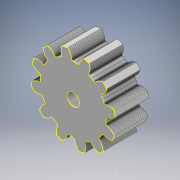
# Autodesk Inventor part: Engranaje_V_P_2
Saved by Autodesk Inventor 2017 (Build 210142000, 142)
## iProperties
Created: 2016-10-02
Part Number: Engranaje_V_P_2
Material: Generic
Document SubType Name: Modeling
Designer: CASA
Density: 1 g/cm^3
Appearance: Default
Author: CASA
Autodesk Inventor part; units mm, degrees
(part 1 of 2)
ref_plane "YZ Plane" through (0, 0, 0) normal (1, 0, 0) x (0, 1, 0)
ref_plane "XZ Plane" through (0, 0, 0) normal (0, 1, 0) x (-1, 0, 0)
ref_plane "XY Plane" through (0, 0, 0) normal (0, 0, 1) x (1, 0, 0)
sketch "Sketch1" plane through (0, 0, 0) normal (0, 1, 0) x (-1, 0, 0)
  line L0 (0.4524, 0.3799) -> (0.4499, 0.3611)
  line L1 (0.4499, 0.3611) -> (0.4427, 0.3436)
  line L2 (0.4427, 0.3436) -> (0.4311, 0.3286)
  line L3 (0.4311, 0.3286) -> (0.4161, 0.3171)
  line L4 (0.4161, 0.3171) -> (0.3986, 0.3099)
  line L5 (0.3986, 0.3099) -> (0.3799, 0.3074)
  line L6 (0.3799, 0.3074) -> (0.3611, 0.3099)
  line L7 (0.3611, 0.3099) -> (0.3436, 0.3171)
  line L8 (0.3436, 0.3171) -> (0.3286, 0.3286)
  line L9 (0.3286, 0.3286) -> (0.3171, 0.3436)
  line L10 (0.3171, 0.3436) -> (0.3099, 0.3611)
  line L11 (0.3099, 0.3611) -> (0.3074, 0.3799)
  line L12 (0.3074, 0.3799) -> (0.3099, 0.3987)
  line L13 (0.3099, 0.3987) -> (0.3171, 0.4161)
  line L14 (0.3171, 0.4161) -> (0.3286, 0.4312)
  line L15 (0.3286, 0.4312) -> (0.3436, 0.4427)
  line L16 (0.3436, 0.4427) -> (0.3611, 0.4499)
  line L17 (0.3611, 0.4499) -> (0.3799, 0.4524)
  line L18 (0.3799, 0.4524) -> (0.3987, 0.4499)
  line L19 (0.3987, 0.4499) -> (0.4161, 0.4427)
  line L20 (0.4161, 0.4427) -> (0.4312, 0.4312)
  line L21 (0.4312, 0.4312) -> (0.4427, 0.4161)
  line L22 (0.4427, 0.4161) -> (0.4499, 0.3987)
  line L23 (0.4499, 0.3987) -> (0.4524, 0.3799)
  line L24 (0.0835, 0.3886) -> (0.0821, 0.3902)
  line L25 (0.0821, 0.3902) -> (0.0807, 0.3913)
  line L26 (0.0807, 0.3913) -> (0.0794, 0.3923)
  line L27 (0.0794, 0.3923) -> (0.078, 0.393)
  line L28 (0.078, 0.393) -> (0.0766, 0.3937)
  line L29 (0.0766, 0.3937) -> (0.0738, 0.3947)
  line L30 (0.0738, 0.3947) -> (0.071, 0.3955)
  line L31 (0.071, 0.3955) -> (0.0682, 0.396)
  line L32 (0.0682, 0.396) -> (0.0626, 0.3967)
  line L33 (0.0626, 0.3967) -> (0.057, 0.3978)
  line L34 (0.057, 0.3978) -> (0.0514, 0.3995)
  line L35 (0.0514, 0.3995) -> (0.0459, 0.4016)
  line L36 (0.0459, 0.4016) -> (0.0404, 0.404)
  line L37 (0.0404, 0.404) -> (0.035, 0.4068)
  line L38 (0.035, 0.4068) -> (0.0295, 0.4098)
  line L39 (0.0295, 0.4098) -> (0.0242, 0.4131)
  line L40 (0.0242, 0.4131) -> (0.0188, 0.4167)
  line L41 (0.0188, 0.4167) -> (0.0136, 0.4206)
  line L42 (0.0136, 0.4206) -> (0.0083, 0.4246)
  line L43 (0.0083, 0.4246) -> (0.0032, 0.4289)
  line L44 (0.0032, 0.4289) -> (0.0136, 0.4806)
  line L45 (0.0136, 0.4806) -> (0.02, 0.4826)
  line L46 (0.02, 0.4826) -> (0.0264, 0.4844)
  line L47 (0.0264, 0.4844) -> (0.0328, 0.4858)
  line L48 (0.0328, 0.4858) -> (0.0391, 0.4871)
  line L49 (0.0391, 0.4871) -> (0.0453, 0.488)
  line L50 (0.0453, 0.488) -> (0.0515, 0.4888)
  line L51 (0.0515, 0.4888) -> (0.0576, 0.4892)
  line L52 (0.0576, 0.4892) -> (0.0636, 0.4893)
  line L53 (0.0636, 0.4893) -> (0.0695, 0.4891)
  line L54 (0.0695, 0.4891) -> (0.0753, 0.4885)
  line L55 (0.0753, 0.4885) -> (0.0809, 0.4873)
  line L56 (0.0809, 0.4873) -> (0.0863, 0.4858)
  line L57 (0.0863, 0.4858) -> (0.0891, 0.4852)
  line L58 (0.0891, 0.4852) -> (0.092, 0.4848)
  line L59 (0.092, 0.4848) -> (0.095, 0.4847)
  line L60 (0.095, 0.4847) -> (0.0965, 0.4848)
  line L61 (0.0965, 0.4848) -> (0.0981, 0.4849)
  line L62 (0.0981, 0.4849) -> (0.0997, 0.4852)
  line L63 (0.0997, 0.4852) -> (0.1014, 0.4858)
  line L64 (0.1014, 0.4858) -> (0.1033, 0.4867)
  line L65 (0.1033, 0.4867) -> (0.106, 0.4899)
  line L66 (0.106, 0.4899) -> (0.1155, 0.5111)
  line L67 (0.1155, 0.5111) -> (0.1267, 0.5315)
  line L68 (0.1267, 0.5315) -> (0.1275, 0.5356)
  line L69 (0.1275, 0.5356) -> (0.1272, 0.5377)
  line L70 (0.1272, 0.5377) -> (0.1265, 0.5394)
  line L71 (0.1265, 0.5394) -> (0.1258, 0.5409)
  line L72 (0.1258, 0.5409) -> (0.125, 0.5422)
  line L73 (0.125, 0.5422) -> (0.1241, 0.5435)
  line L74 (0.1241, 0.5435) -> (0.1222, 0.5457)
  line L75 (0.1222, 0.5457) -> (0.1202, 0.5478)
  line L76 (0.1202, 0.5478) -> (0.1181, 0.5497)
  line L77 (0.1181, 0.5497) -> (0.1135, 0.5531)
  line L78 (0.1135, 0.5531) -> (0.1092, 0.5568)
  line L79 (0.1092, 0.5568) -> (0.1052, 0.5611)
  line L80 (0.1052, 0.5611) -> (0.1015, 0.5657)
  line L81 (0.1015, 0.5657) -> (0.098, 0.5705)
  line L82 (0.098, 0.5705) -> (0.0946, 0.5756)
  line L83 (0.0946, 0.5756) -> (0.0914, 0.581)
  line L84 (0.0914, 0.581) -> (0.0884, 0.5866)
  line L85 (0.0884, 0.5866) -> (0.0856, 0.5923)
  line L86 (0.0856, 0.5923) -> (0.083, 0.5983)
  line L87 (0.083, 0.5983) -> (0.0805, 0.6044)
  line L88 (0.0805, 0.6044) -> (0.0782, 0.6107)
  line L89 (0.0782, 0.6107) -> (0.1131, 0.6503)
  line L90 (0.1131, 0.6503) -> (0.1196, 0.6488)
  line L91 (0.1196, 0.6488) -> (0.126, 0.6471)
  line L92 (0.126, 0.6471) -> (0.1323, 0.6452)
  line L93 (0.1323, 0.6452) -> (0.1383, 0.6431)
  line L94 (0.1383, 0.6431) -> (0.1442, 0.6409)
  line L95 (0.1442, 0.6409) -> (0.1499, 0.6384)
  line L96 (0.1499, 0.6384) -> (0.1554, 0.6357)
  line L97 (0.1554, 0.6357) -> (0.1607, 0.6328)
  line L98 (0.1607, 0.6328) -> (0.1657, 0.6296)
  line L99 (0.1657, 0.6296) -> (0.1704, 0.6262)
  line L100 (0.1704, 0.6262) -> (0.1747, 0.6224)
  line L101 (0.1747, 0.6224) -> (0.1786, 0.6184)
  line L102 (0.1786, 0.6184) -> (0.1807, 0.6165)
  line L103 (0.1807, 0.6165) -> (0.183, 0.6147)
  line L104 (0.183, 0.6147) -> (0.1855, 0.6131)
  line L105 (0.1855, 0.6131) -> (0.1869, 0.6124)
  line L106 (0.1869, 0.6124) -> (0.1883, 0.6118)
  line L107 (0.1883, 0.6118) -> (0.1899, 0.6112)
  line L108 (0.1899, 0.6112) -> (0.1917, 0.6108)
  line L109 (0.1917, 0.6108) -> (0.1937, 0.6107)
  line L110 (0.1937, 0.6107) -> (0.1978, 0.6121)
  line L111 (0.1978, 0.6121) -> (0.2166, 0.6257)
  line L112 (0.2166, 0.6257) -> (0.2364, 0.6378)
  line L113 (0.2364, 0.6378) -> (0.2392, 0.6409)
  line L114 (0.2392, 0.6409) -> (0.2399, 0.6429)
  line L115 (0.2399, 0.6429) -> (0.2402, 0.6447)
  line L116 (0.2402, 0.6447) -> (0.2403, 0.6463)
  line L117 (0.2403, 0.6463) -> (0.2403, 0.6479)
  line L118 (0.2403, 0.6479) -> (0.2402, 0.6494)
  line L119 (0.2402, 0.6494) -> (0.2397, 0.6524)
  line L120 (0.2397, 0.6524) -> (0.2389, 0.6552)
  line L121 (0.2389, 0.6552) -> (0.238, 0.6579)
  line L122 (0.238, 0.6579) -> (0.2358, 0.6631)
  line L123 (0.2358, 0.6631) -> (0.234, 0.6685)
  line L124 (0.234, 0.6685) -> (0.2326, 0.6741)
  line L125 (0.2326, 0.6741) -> (0.2317, 0.68)
  line L126 (0.2317, 0.68) -> (0.2311, 0.6859)
  line L127 (0.2311, 0.6859) -> (0.2307, 0.6921)
  line L128 (0.2307, 0.6921) -> (0.2306, 0.6983)
  line L129 (0.2306, 0.6983) -> (0.2308, 0.7046)
  line L130 (0.2308, 0.7046) -> (0.2312, 0.711)
  line L131 (0.2312, 0.711) -> (0.2319, 0.7175)
  line L132 (0.2319, 0.7175) -> (0.2328, 0.724)
  line L133 (0.2328, 0.724) -> (0.234, 0.7306)
  line L134 (0.234, 0.7306) -> (0.284, 0.7475)
  line L135 (0.284, 0.7475) -> (0.2889, 0.7429)
  line L136 (0.2889, 0.7429) -> (0.2936, 0.7382)
  line L137 (0.2936, 0.7382) -> (0.2981, 0.7335)
  line L138 (0.2981, 0.7335) -> (0.3023, 0.7286)
  line L139 (0.3023, 0.7286) -> (0.3063, 0.7237)
  line L140 (0.3063, 0.7237) -> (0.31, 0.7187)
  line L141 (0.31, 0.7187) -> (0.3134, 0.7137)
  line L142 (0.3134, 0.7137) -> (0.3165, 0.7085)
  line L143 (0.3165, 0.7085) -> (0.3193, 0.7033)
  line L144 (0.3193, 0.7033) -> (0.3216, 0.698)
  line L145 (0.3216, 0.698) -> (0.3234, 0.6926)
  line L146 (0.3234, 0.6926) -> (0.3248, 0.6871)
  line L147 (0.3248, 0.6871) -> (0.3257, 0.6844)
  line L148 (0.3257, 0.6844) -> (0.3268, 0.6817)
  line L149 (0.3268, 0.6817) -> (0.3282, 0.6791)
  line L150 (0.3282, 0.6791) -> (0.329, 0.6778)
  line L151 (0.329, 0.6778) -> (0.3299, 0.6765)
  line L152 (0.3299, 0.6765) -> (0.331, 0.6752)
  line L153 (0.331, 0.6752) -> (0.3323, 0.674)
  line L154 (0.3323, 0.674) -> (0.3341, 0.6729)
  line L155 (0.3341, 0.6729) -> (0.3382, 0.6721)
  line L156 (0.3382, 0.6721) -> (0.3613, 0.6744)
  line L157 (0.3613, 0.6744) -> (0.3846, 0.675)
  line L158 (0.3846, 0.675) -> (0.3886, 0.6763)
  line L159 (0.3886, 0.6763) -> (0.3902, 0.6777)
  line L160 (0.3902, 0.6777) -> (0.3913, 0.679)
  line L161 (0.3913, 0.679) -> (0.3923, 0.6804)
  line L162 (0.3923, 0.6804) -> (0.393, 0.6818)
  line L163 (0.393, 0.6818) -> (0.3937, 0.6832)
  line L164 (0.3937, 0.6832) -> (0.3947, 0.686)
  line L165 (0.3947, 0.686) -> (0.3955, 0.6887)
  line L166 (0.3955, 0.6887) -> (0.396, 0.6915)
  line L167 (0.396, 0.6915) -> (0.3967, 0.6972)
  line L168 (0.3967, 0.6972) -> (0.3978, 0.7028)
  line L169 (0.3978, 0.7028) -> (0.3995, 0.7083)
  line L170 (0.3995, 0.7083) -> (0.4016, 0.7139)
  line L171 (0.4016, 0.7139) -> (0.404, 0.7194)
  line L172 (0.404, 0.7194) -> (0.4068, 0.7248)
  line L173 (0.4068, 0.7248) -> (0.4098, 0.7302)
  line L174 (0.4098, 0.7302) -> (0.4131, 0.7356)
  line L175 (0.4131, 0.7356) -> (0.4167, 0.7409)
  line L176 (0.4167, 0.7409) -> (0.4205, 0.7462)
  line L177 (0.4205, 0.7462) -> (0.4246, 0.7514)
  line L178 (0.4246, 0.7514) -> (0.4289, 0.7566)
  line L179 (0.4289, 0.7566) -> (0.4806, 0.7462)
  line L180 (0.4806, 0.7462) -> (0.4826, 0.7397)
  line L181 (0.4826, 0.7397) -> (0.4843, 0.7334)
  line L182 (0.4843, 0.7334) -> (0.4858, 0.727)
  line L183 (0.4858, 0.727) -> (0.4871, 0.7207)
  line L184 (0.4871, 0.7207) -> (0.488, 0.7145)
  line L185 (0.488, 0.7145) -> (0.4887, 0.7083)
  line L186 (0.4887, 0.7083) -> (0.4892, 0.7022)
  line L187 (0.4892, 0.7022) -> (0.4893, 0.6962)
  line L188 (0.4893, 0.6962) -> (0.4891, 0.6903)
  line L189 (0.4891, 0.6903) -> (0.4885, 0.6845)
  line L190 (0.4885, 0.6845) -> (0.4873, 0.6789)
  line L191 (0.4873, 0.6789) -> (0.4858, 0.6734)
  line L192 (0.4858, 0.6734) -> (0.4852, 0.6706)
  line L193 (0.4852, 0.6706) -> (0.4848, 0.6678)
  line L194 (0.4848, 0.6678) -> (0.4847, 0.6648)
  line L195 (0.4847, 0.6648) -> (0.4848, 0.6633)
  line L196 (0.4848, 0.6633) -> (0.4849, 0.6617)
  line L197 (0.4849, 0.6617) -> (0.4852, 0.6601)
  line L198 (0.4852, 0.6601) -> (0.4858, 0.6584)
  line L199 (0.4858, 0.6584) -> (0.4867, 0.6565)
  line L200 (0.4867, 0.6565) -> (0.4899, 0.6537)
  line L201 (0.4899, 0.6537) -> (0.5111, 0.6442)
  line L202 (0.5111, 0.6442) -> (0.5315, 0.6331)
  line L203 (0.5315, 0.6331) -> (0.5356, 0.6322)
  line L204 (0.5356, 0.6322) -> (0.5377, 0.6326)
  line L205 (0.5377, 0.6326) -> (0.5394, 0.6332)
  line L206 (0.5394, 0.6332) -> (0.5409, 0.634)
  line L207 (0.5409, 0.634) -> (0.5422, 0.6348)
  line L208 (0.5422, 0.6348) -> (0.5435, 0.6356)
  line L209 (0.5435, 0.6356) -> (0.5457, 0.6375)
  line L210 (0.5457, 0.6375) -> (0.5478, 0.6396)
  line L211 (0.5478, 0.6396) -> (0.5497, 0.6417)
  line L212 (0.5497, 0.6417) -> (0.5531, 0.6463)
  line L213 (0.5531, 0.6463) -> (0.5568, 0.6505)
  line L214 (0.5568, 0.6505) -> (0.5611, 0.6545)
  line L215 (0.5611, 0.6545) -> (0.5657, 0.6583)
  line L216 (0.5657, 0.6583) -> (0.5705, 0.6618)
  line L217 (0.5705, 0.6618) -> (0.5756, 0.6652)
  line L218 (0.5756, 0.6652) -> (0.581, 0.6683)
  line L219 (0.581, 0.6683) -> (0.5865, 0.6713)
  line L220 (0.5865, 0.6713) -> (0.5923, 0.6742)
  line L221 (0.5923, 0.6742) -> (0.5983, 0.6768)
  line L222 (0.5983, 0.6768) -> (0.6044, 0.6793)
  line L223 (0.6044, 0.6793) -> (0.6107, 0.6816)
  line L224 (0.6107, 0.6816) -> (0.6503, 0.6467)
  line L225 (0.6503, 0.6467) -> (0.6488, 0.6402)
  line L226 (0.6488, 0.6402) -> (0.6471, 0.6338)
  line L227 (0.6471, 0.6338) -> (0.6452, 0.6275)
  line L228 (0.6452, 0.6275) -> (0.6431, 0.6214)
  line L229 (0.6431, 0.6214) -> (0.6408, 0.6156)
  line L230 (0.6408, 0.6156) -> (0.6384, 0.6099)
  line L231 (0.6384, 0.6099) -> (0.6357, 0.6044)
  line L232 (0.6357, 0.6044) -> (0.6328, 0.5991)
  line L233 (0.6328, 0.5991) -> (0.6296, 0.5941)
  line L234 (0.6296, 0.5941) -> (0.6262, 0.5894)
  line L235 (0.6262, 0.5894) -> (0.6224, 0.5851)
  line L236 (0.6224, 0.5851) -> (0.6184, 0.5812)
  line L237 (0.6184, 0.5812) -> (0.6165, 0.579)
  line L238 (0.6165, 0.579) -> (0.6147, 0.5767)
  line L239 (0.6147, 0.5767) -> (0.6131, 0.5742)
  line L240 (0.6131, 0.5742) -> (0.6124, 0.5729)
  line L241 (0.6124, 0.5729) -> (0.6118, 0.5714)
  line L242 (0.6118, 0.5714) -> (0.6112, 0.5699)
  line L243 (0.6112, 0.5699) -> (0.6108, 0.5681)
  line L244 (0.6108, 0.5681) -> (0.6107, 0.566)
  line L245 (0.6107, 0.566) -> (0.6121, 0.562)
  line L246 (0.6121, 0.562) -> (0.6257, 0.5432)
  line L247 (0.6257, 0.5432) -> (0.6378, 0.5234)
  line L248 (0.6378, 0.5234) -> (0.6409, 0.5205)
  line L249 (0.6409, 0.5205) -> (0.6429, 0.5198)
  line L250 (0.6429, 0.5198) -> (0.6447, 0.5195)
  line L251 (0.6447, 0.5195) -> (0.6463, 0.5194)
  line L252 (0.6463, 0.5194) -> (0.6479, 0.5195)
  line L253 (0.6479, 0.5195) -> (0.6494, 0.5196)
  line L254 (0.6494, 0.5196) -> (0.6523, 0.5201)
  line L255 (0.6523, 0.5201) -> (0.6551, 0.5208)
  line L256 (0.6551, 0.5208) -> (0.6578, 0.5217)
  line L257 (0.6578, 0.5217) -> (0.6631, 0.524)
  line L258 (0.6631, 0.524) -> (0.6685, 0.5258)
  line L259 (0.6685, 0.5258) -> (0.6741, 0.5271)
  line L260 (0.6741, 0.5271) -> (0.68, 0.5281)
  line L261 (0.68, 0.5281) -> (0.6859, 0.5287)
  line L262 (0.6859, 0.5287) -> (0.692, 0.5291)
  line L263 (0.692, 0.5291) -> (0.6983, 0.5291)
  line L264 (0.6983, 0.5291) -> (0.7046, 0.529)
  line L265 (0.7046, 0.529) -> (0.711, 0.5285)
  line L266 (0.711, 0.5285) -> (0.7175, 0.5278)
  line L267 (0.7175, 0.5278) -> (0.724, 0.5269)
  line L268 (0.724, 0.5269) -> (0.7306, 0.5258)
  line L269 (0.7306, 0.5258) -> (0.7475, 0.4758)
  line L270 (0.7475, 0.4758) -> (0.7429, 0.4708)
  line L271 (0.7429, 0.4708) -> (0.7382, 0.4661)
  line L272 (0.7382, 0.4661) -> (0.7335, 0.4617)
  line L273 (0.7335, 0.4617) -> (0.7286, 0.4575)
  line L274 (0.7286, 0.4575) -> (0.7237, 0.4535)
  line L275 (0.7237, 0.4535) -> (0.7187, 0.4498)
  line L276 (0.7187, 0.4498) -> (0.7137, 0.4464)
  line L277 (0.7137, 0.4464) -> (0.7085, 0.4433)
  line L278 (0.7085, 0.4433) -> (0.7033, 0.4405)
  line L279 (0.7033, 0.4405) -> (0.698, 0.4381)
  line L280 (0.698, 0.4381) -> (0.6926, 0.4363)
  line L281 (0.6926, 0.4363) -> (0.6871, 0.4349)
  line L282 (0.6871, 0.4349) -> (0.6844, 0.434)
  line L283 (0.6844, 0.434) -> (0.6817, 0.4329)
  line L284 (0.6817, 0.4329) -> (0.6791, 0.4316)
  line L285 (0.6791, 0.4316) -> (0.6778, 0.4308)
  line L286 (0.6778, 0.4308) -> (0.6765, 0.4298)
  line L287 (0.6765, 0.4298) -> (0.6752, 0.4287)
  line L288 (0.6752, 0.4287) -> (0.674, 0.4274)
  line L289 (0.674, 0.4274) -> (0.6729, 0.4257)
  line L290 (0.6729, 0.4257) -> (0.6721, 0.4215)
  line L291 (0.6721, 0.4215) -> (0.6744, 0.3984)
  line L292 (0.6744, 0.3984) -> (0.675, 0.3752)
  line L293 (0.675, 0.3752) -> (0.6763, 0.3712)
  line L294 (0.6763, 0.3712) -> (0.6777, 0.3696)
  line L295 (0.6777, 0.3696) -> (0.679, 0.3684)
  line L296 (0.679, 0.3684) -> (0.6804, 0.3675)
  line L297 (0.6804, 0.3675) -> (0.6818, 0.3667)
  line L298 (0.6818, 0.3667) -> (0.6832, 0.3661)
  line L299 (0.6832, 0.3661) -> (0.686, 0.3651)
  line L300 (0.686, 0.3651) -> (0.6887, 0.3643)
  line L301 (0.6887, 0.3643) -> (0.6915, 0.3637)
  line L302 (0.6915, 0.3637) -> (0.6972, 0.3631)
  line L303 (0.6972, 0.3631) -> (0.7028, 0.3619)
  line L304 (0.7028, 0.3619) -> (0.7083, 0.3603)
  line L305 (0.7083, 0.3603) -> (0.7139, 0.3582)
  line L306 (0.7139, 0.3582) -> (0.7194, 0.3557)
  line L307 (0.7194, 0.3557) -> (0.7248, 0.353)
  line L308 (0.7248, 0.353) -> (0.7302, 0.3499)
  line L309 (0.7302, 0.3499) -> (0.7356, 0.3466)
  line L310 (0.7356, 0.3466) -> (0.7409, 0.343)
  line L311 (0.7409, 0.343) -> (0.7462, 0.3392)
  line L312 (0.7462, 0.3392) -> (0.7514, 0.3351)
  line L313 (0.7514, 0.3351) -> (0.7566, 0.3308)
  line L314 (0.7566, 0.3308) -> (0.7462, 0.2791)
  line L315 (0.7462, 0.2791) -> (0.7397, 0.2771)
  line L316 (0.7397, 0.2771) -> (0.7334, 0.2754)
  line L317 (0.7334, 0.2754) -> (0.727, 0.2739)
  line L318 (0.727, 0.2739) -> (0.7207, 0.2727)
  line L319 (0.7207, 0.2727) -> (0.7145, 0.2717)
  line L320 (0.7145, 0.2717) -> (0.7083, 0.271)
  line L321 (0.7083, 0.271) -> (0.7022, 0.2706)
  line L322 (0.7022, 0.2706) -> (0.6962, 0.2705)
  line L323 (0.6962, 0.2705) -> (0.6903, 0.2707)
  line L324 (0.6903, 0.2707) -> (0.6845, 0.2713)
  line L325 (0.6845, 0.2713) -> (0.6789, 0.2724)
  line L326 (0.6789, 0.2724) -> (0.6734, 0.274)
  line L327 (0.6734, 0.274) -> (0.6706, 0.2746)
  line L328 (0.6706, 0.2746) -> (0.6678, 0.2749)
  line L329 (0.6678, 0.2749) -> (0.6648, 0.2751)
  line L330 (0.6648, 0.2751) -> (0.6633, 0.275)
  line L331 (0.6633, 0.275) -> (0.6617, 0.2748)
  line L332 (0.6617, 0.2748) -> (0.6601, 0.2745)
  line L333 (0.6601, 0.2745) -> (0.6584, 0.274)
  line L334 (0.6584, 0.274) -> (0.6565, 0.2731)
  line L335 (0.6565, 0.2731) -> (0.6537, 0.2699)
  line L336 (0.6537, 0.2699) -> (0.6442, 0.2487)
  line L337 (0.6442, 0.2487) -> (0.6331, 0.2283)
  line L338 (0.6331, 0.2283) -> (0.6322, 0.2241)
  line L339 (0.6322, 0.2241) -> (0.6326, 0.2221)
  line L340 (0.6326, 0.2221) -> (0.6332, 0.2204)
  line L341 (0.6332, 0.2204) -> (0.634, 0.2189)
  line L342 (0.634, 0.2189) -> (0.6348, 0.2176)
  line L343 (0.6348, 0.2176) -> (0.6356, 0.2163)
  line L344 (0.6356, 0.2163) -> (0.6375, 0.214)
  line L345 (0.6375, 0.214) -> (0.6396, 0.212)
  line L346 (0.6396, 0.212) -> (0.6417, 0.2101)
  line L347 (0.6417, 0.2101) -> (0.6463, 0.2067)
  line L348 (0.6463, 0.2067) -> (0.6505, 0.2029)
  line L349 (0.6505, 0.2029) -> (0.6545, 0.1987)
  line L350 (0.6545, 0.1987) -> (0.6583, 0.1941)
  line L351 (0.6583, 0.1941) -> (0.6618, 0.1892)
  line L352 (0.6618, 0.1892) -> (0.6652, 0.1841)
  line L353 (0.6652, 0.1841) -> (0.6683, 0.1788)
  line L354 (0.6683, 0.1788) -> (0.6713, 0.1732)
  line L355 (0.6713, 0.1732) -> (0.6742, 0.1675)
  line L356 (0.6742, 0.1675) -> (0.6768, 0.1615)
  line L357 (0.6768, 0.1615) -> (0.6793, 0.1554)
  line L358 (0.6793, 0.1554) -> (0.6816, 0.1491)
  line L359 (0.6816, 0.1491) -> (0.6467, 0.1095)
  line L360 (0.6467, 0.1095) -> (0.6402, 0.111)
  line L361 (0.6402, 0.111) -> (0.6338, 0.1127)
  line L362 (0.6338, 0.1127) -> (0.6275, 0.1146)
  line L363 (0.6275, 0.1146) -> (0.6214, 0.1166)
  line L364 (0.6214, 0.1166) -> (0.6156, 0.1189)
  line L365 (0.6156, 0.1189) -> (0.6099, 0.1214)
  line L366 (0.6099, 0.1214) -> (0.6044, 0.1241)
  line L367 (0.6044, 0.1241) -> (0.5991, 0.127)
  line L368 (0.5991, 0.127) -> (0.5941, 0.1301)
  line L369 (0.5941, 0.1301) -> (0.5894, 0.1335)
  line L370 (0.5894, 0.1335) -> (0.5851, 0.1373)
  line L371 (0.5851, 0.1373) -> (0.5812, 0.1414)
  line L372 (0.5812, 0.1414) -> (0.579, 0.1433)
  line L373 (0.579, 0.1433) -> (0.5767, 0.145)
  line L374 (0.5767, 0.145) -> (0.5742, 0.1466)
  line L375 (0.5742, 0.1466) -> (0.5729, 0.1474)
  line L376 (0.5729, 0.1474) -> (0.5714, 0.148)
  line L377 (0.5714, 0.148) -> (0.5699, 0.1485)
  line L378 (0.5699, 0.1485) -> (0.5681, 0.1489)
  line L379 (0.5681, 0.1489) -> (0.566, 0.1491)
  line L380 (0.566, 0.1491) -> (0.562, 0.1477)
  line L381 (0.562, 0.1477) -> (0.5432, 0.1341)
  line L382 (0.5432, 0.1341) -> (0.5234, 0.122)
  line L383 (0.5234, 0.122) -> (0.5205, 0.1188)
  line L384 (0.5205, 0.1188) -> (0.5198, 0.1169)
  line L385 (0.5198, 0.1169) -> (0.5195, 0.1151)
  line L386 (0.5195, 0.1151) -> (0.5194, 0.1134)
  line L387 (0.5194, 0.1134) -> (0.5194, 0.1119)
  line L388 (0.5194, 0.1119) -> (0.5196, 0.1103)
  line L389 (0.5196, 0.1103) -> (0.5201, 0.1074)
  line L390 (0.5201, 0.1074) -> (0.5208, 0.1046)
  line L391 (0.5208, 0.1046) -> (0.5217, 0.1019)
  line L392 (0.5217, 0.1019) -> (0.524, 0.0967)
  line L393 (0.524, 0.0967) -> (0.5258, 0.0913)
  line L394 (0.5258, 0.0913) -> (0.5271, 0.0856)
  line L395 (0.5271, 0.0856) -> (0.5281, 0.0798)
  line L396 (0.5281, 0.0798) -> (0.5287, 0.0738)
  line L397 (0.5287, 0.0738) -> (0.5291, 0.0677)
  line L398 (0.5291, 0.0677) -> (0.5291, 0.0615)
  line L399 (0.5291, 0.0615) -> (0.529, 0.0552)
  line L400 (0.529, 0.0552) -> (0.5285, 0.0488)
  line L401 (0.5285, 0.0488) -> (0.5278, 0.0423)
  line L402 (0.5278, 0.0423) -> (0.5269, 0.0357)
  line L403 (0.5269, 0.0357) -> (0.5258, 0.0291)
  line L404 (0.5258, 0.0291) -> (0.4758, 0.0123)
  line L405 (0.4758, 0.0123) -> (0.4708, 0.0169)
  line L406 (0.4708, 0.0169) -> (0.4661, 0.0215)
  line L407 (0.4661, 0.0215) -> (0.4617, 0.0263)
  line L408 (0.4617, 0.0263) -> (0.4575, 0.0311)
  line L409 (0.4575, 0.0311) -> (0.4535, 0.036)
  line L410 (0.4535, 0.036) -> (0.4498, 0.041)
  line L411 (0.4498, 0.041) -> (0.4464, 0.0461)
  line L412 (0.4464, 0.0461) -> (0.4433, 0.0513)
  line L413 (0.4433, 0.0513) -> (0.4405, 0.0565)
  line L414 (0.4405, 0.0565) -> (0.4381, 0.0618)
  line L415 (0.4381, 0.0618) -> (0.4363, 0.0672)
  line L416 (0.4363, 0.0672) -> (0.435, 0.0727)
  line L417 (0.435, 0.0727) -> (0.4341, 0.0754)
  line L418 (0.4341, 0.0754) -> (0.4329, 0.0781)
  line L419 (0.4329, 0.0781) -> (0.4316, 0.0807)
  line L420 (0.4316, 0.0807) -> (0.4308, 0.082)
  line L421 (0.4308, 0.082) -> (0.4298, 0.0833)
  line L422 (0.4298, 0.0833) -> (0.4287, 0.0845)
  line L423 (0.4287, 0.0845) -> (0.4274, 0.0858)
  line L424 (0.4274, 0.0858) -> (0.4257, 0.0869)
  line L425 (0.4257, 0.0869) -> (0.4215, 0.0877)
  line L426 (0.4215, 0.0877) -> (0.3984, 0.0853)
  line L427 (0.3984, 0.0853) -> (0.3752, 0.0848)
  line L428 (0.3752, 0.0848) -> (0.3712, 0.0835)
  line L429 (0.3712, 0.0835) -> (0.3696, 0.0821)
  line L430 (0.3696, 0.0821) -> (0.3684, 0.0807)
  line L431 (0.3684, 0.0807) -> (0.3675, 0.0794)
  line L432 (0.3675, 0.0794) -> (0.3667, 0.078)
  line L433 (0.3667, 0.078) -> (0.3661, 0.0766)
  line L434 (0.3661, 0.0766) -> (0.3651, 0.0738)
  line L435 (0.3651, 0.0738) -> (0.3643, 0.071)
  line L436 (0.3643, 0.071) -> (0.3638, 0.0682)
  line L437 (0.3638, 0.0682) -> (0.3631, 0.0626)
  line L438 (0.3631, 0.0626) -> (0.362, 0.057)
  line L439 (0.362, 0.057) -> (0.3603, 0.0514)
  line L440 (0.3603, 0.0514) -> (0.3582, 0.0459)
  line L441 (0.3582, 0.0459) -> (0.3557, 0.0404)
  line L442 (0.3557, 0.0404) -> (0.353, 0.0349)
  line L443 (0.353, 0.0349) -> (0.3499, 0.0295)
  line L444 (0.3499, 0.0295) -> (0.3466, 0.0241)
  line L445 (0.3466, 0.0241) -> (0.3431, 0.0188)
  line L446 (0.3431, 0.0188) -> (0.3392, 0.0135)
  line L447 (0.3392, 0.0135) -> (0.3351, 0.0083)
  line L448 (0.3351, 0.0083) -> (0.3308, 0.0032)
  line L449 (0.3308, 0.0032) -> (0.2791, 0.0136)
  line L450 (0.2791, 0.0136) -> (0.2771, 0.02)
  line L451 (0.2771, 0.02) -> (0.2754, 0.0264)
  line L452 (0.2754, 0.0264) -> (0.2739, 0.0328)
  line L453 (0.2739, 0.0328) -> (0.2727, 0.0391)
  line L454 (0.2727, 0.0391) -> (0.2717, 0.0453)
  line L455 (0.2717, 0.0453) -> (0.271, 0.0515)
  line L456 (0.271, 0.0515) -> (0.2706, 0.0576)
  line L457 (0.2706, 0.0576) -> (0.2705, 0.0636)
  line L458 (0.2705, 0.0636) -> (0.2707, 0.0695)
  line L459 (0.2707, 0.0695) -> (0.2713, 0.0753)
  line L460 (0.2713, 0.0753) -> (0.2724, 0.0809)
  line L461 (0.2724, 0.0809) -> (0.274, 0.0863)
  line L462 (0.274, 0.0863) -> (0.2746, 0.0891)
  line L463 (0.2746, 0.0891) -> (0.2749, 0.092)
  line L464 (0.2749, 0.092) -> (0.2751, 0.0949)
  line L465 (0.2751, 0.0949) -> (0.275, 0.0965)
  line L466 (0.275, 0.0965) -> (0.2748, 0.098)
  line L467 (0.2748, 0.098) -> (0.2745, 0.0997)
  line L468 (0.2745, 0.0997) -> (0.274, 0.1014)
  line L469 (0.274, 0.1014) -> (0.2731, 0.1033)
  line L470 (0.2731, 0.1033) -> (0.2699, 0.106)
  line L471 (0.2699, 0.106) -> (0.2487, 0.1155)
  line L472 (0.2487, 0.1155) -> (0.2283, 0.1267)
  line L473 (0.2283, 0.1267) -> (0.2241, 0.1276)
  line L474 (0.2241, 0.1276) -> (0.2221, 0.1272)
  line L475 (0.2221, 0.1272) -> (0.2204, 0.1266)
  line L476 (0.2204, 0.1266) -> (0.2189, 0.1258)
  line L477 (0.2189, 0.1258) -> (0.2176, 0.125)
  line L478 (0.2176, 0.125) -> (0.2163, 0.1241)
  line L479 (0.2163, 0.1241) -> (0.214, 0.1222)
  line L480 (0.214, 0.1222) -> (0.212, 0.1202)
  line L481 (0.212, 0.1202) -> (0.2101, 0.1181)
  line L482 (0.2101, 0.1181) -> (0.2067, 0.1135)
  line L483 (0.2067, 0.1135) -> (0.2029, 0.1092)
  line L484 (0.2029, 0.1092) -> (0.1987, 0.1053)
  line L485 (0.1987, 0.1053) -> (0.1941, 0.1015)
  line L486 (0.1941, 0.1015) -> (0.1892, 0.098)
  line L487 (0.1892, 0.098) -> (0.1841, 0.0946)
  line L488 (0.1841, 0.0946) -> (0.1788, 0.0914)
  line L489 (0.1788, 0.0914) -> (0.1732, 0.0884)
  line L490 (0.1732, 0.0884) -> (0.1675, 0.0856)
  line L491 (0.1675, 0.0856) -> (0.1615, 0.083)
  line L492 (0.1615, 0.083) -> (0.1554, 0.0805)
  line L493 (0.1554, 0.0805) -> (0.1491, 0.0782)
  line L494 (0.1491, 0.0782) -> (0.1095, 0.1131)
  line L495 (0.1095, 0.1131) -> (0.111, 0.1196)
  line L496 (0.111, 0.1196) -> (0.1127, 0.126)
  line L497 (0.1127, 0.126) -> (0.1146, 0.1323)
  line L498 (0.1146, 0.1323) -> (0.1166, 0.1383)
  line L499 (0.1166, 0.1383) -> (0.1189, 0.1442)
  line L500 (0.1189, 0.1442) -> (0.1214, 0.1499)
  line L501 (0.1214, 0.1499) -> (0.1241, 0.1554)
  line L502 (0.1241, 0.1554) -> (0.127, 0.1607)
  line L503 (0.127, 0.1607) -> (0.1301, 0.1657)
  line L504 (0.1301, 0.1657) -> (0.1335, 0.1704)
  line L505 (0.1335, 0.1704) -> (0.1373, 0.1747)
  line L506 (0.1373, 0.1747) -> (0.1414, 0.1786)
  line L507 (0.1414, 0.1786) -> (0.1433, 0.1807)
  line L508 (0.1433, 0.1807) -> (0.1451, 0.183)
  line L509 (0.1451, 0.183) -> (0.1466, 0.1855)
  line L510 (0.1466, 0.1855) -> (0.1474, 0.1869)
  line L511 (0.1474, 0.1869) -> (0.148, 0.1883)
  line L512 (0.148, 0.1883) -> (0.1485, 0.1899)
  line L513 (0.1485, 0.1899) -> (0.1489, 0.1917)
  line L514 (0.1489, 0.1917) -> (0.1491, 0.1937)
  line L515 (0.1491, 0.1937) -> (0.1477, 0.1978)
  line L516 (0.1477, 0.1978) -> (0.1341, 0.2166)
  line L517 (0.1341, 0.2166) -> (0.122, 0.2364)
  line L518 (0.122, 0.2364) -> (0.1188, 0.2392)
  line L519 (0.1188, 0.2392) -> (0.1169, 0.2399)
  line L520 (0.1169, 0.2399) -> (0.1151, 0.2402)
  line L521 (0.1151, 0.2402) -> (0.1134, 0.2403)
  line L522 (0.1134, 0.2403) -> (0.1119, 0.2403)
  line L523 (0.1119, 0.2403) -> (0.1103, 0.2402)
  line L524 (0.1103, 0.2402) -> (0.1074, 0.2397)
  line L525 (0.1074, 0.2397) -> (0.1046, 0.239)
  line L526 (0.1046, 0.239) -> (0.1019, 0.238)
  line L527 (0.1019, 0.238) -> (0.0967, 0.2358)
  line L528 (0.0967, 0.2358) -> (0.0913, 0.234)
  line L529 (0.0913, 0.234) -> (0.0856, 0.2327)
  line L530 (0.0856, 0.2327) -> (0.0798, 0.2317)
  line L531 (0.0798, 0.2317) -> (0.0738, 0.2311)
  line L532 (0.0738, 0.2311) -> (0.0677, 0.2307)
  line L533 (0.0677, 0.2307) -> (0.0615, 0.2306)
  line L534 (0.0615, 0.2306) -> (0.0552, 0.2308)
  line L535 (0.0552, 0.2308) -> (0.0488, 0.2313)
  line L536 (0.0488, 0.2313) -> (0.0423, 0.2319)
  line L537 (0.0423, 0.2319) -> (0.0357, 0.2329)
  line L538 (0.0357, 0.2329) -> (0.0291, 0.234)
  line L539 (0.0291, 0.234) -> (0.0123, 0.284)
  line L540 (0.0123, 0.284) -> (0.0169, 0.2889)
  line L541 (0.0169, 0.2889) -> (0.0215, 0.2936)
  line L542 (0.0215, 0.2936) -> (0.0263, 0.2981)
  line L543 (0.0263, 0.2981) -> (0.0311, 0.3023)
  line L544 (0.0311, 0.3023) -> (0.036, 0.3063)
  line L545 (0.036, 0.3063) -> (0.041, 0.31)
  line L546 (0.041, 0.31) -> (0.0461, 0.3134)
  line L547 (0.0461, 0.3134) -> (0.0513, 0.3165)
  line L548 (0.0513, 0.3165) -> (0.0565, 0.3193)
  line L549 (0.0565, 0.3193) -> (0.0618, 0.3216)
  line L550 (0.0618, 0.3216) -> (0.0672, 0.3234)
  line L551 (0.0672, 0.3234) -> (0.0727, 0.3248)
  line L552 (0.0727, 0.3248) -> (0.0754, 0.3257)
  line L553 (0.0754, 0.3257) -> (0.0781, 0.3268)
  line L554 (0.0781, 0.3268) -> (0.0807, 0.3282)
  line L555 (0.0807, 0.3282) -> (0.082, 0.329)
  line L556 (0.082, 0.329) -> (0.0833, 0.3299)
  line L557 (0.0833, 0.3299) -> (0.0845, 0.331)
  line L558 (0.0845, 0.331) -> (0.0858, 0.3323)
  line L559 (0.0858, 0.3323) -> (0.0869, 0.3341)
  line L560 (0.0869, 0.3341) -> (0.0877, 0.3382)
  line L561 (0.0877, 0.3382) -> (0.0853, 0.3614)
  line L562 (0.0853, 0.3614) -> (0.0848, 0.3846)
  line L563 (0.0848, 0.3846) -> (0.0835, 0.3886)
  circle A0 centre (0.3799, 0.3799) radius 0.057
  point P0 (0, 0)
  dimension "d2" = 0.114
  constraints: 1128 end point, 211 perpendicular, 50 parallel, 1 centre point, 3 other
  measures "d2" diameter of A0
extrude "Extrusion1" add sketch "Sketch1" along normal blind 0.3 contours L0 L1 L2 L3 L4 L5 L6 L7 L8 L9 L10 L11 L12 L13 L14 L15 L16 L17 L18 L19 L20 L21 L22 L23 | L25 L27 L29 L30 L31 L32 L33 L34 L35 L36 L37 L38 L39 L40 L41 L42 L43 L44 L45 L46 L47 L48 L49 L50 L51 L52 L53 L54 L55 L56 L57 L58 L59 L61 L63 L65 L66 L67 L68 L69 L71 L73 L74 L75 L76 L77 L78 L79 L80 L81 L82 L83 L84 L85 L86 L87 L88 L89 L90 L91 L92 L93 L94 L95 L96 L97 L98 L99 L100 L101 L102 L103 L104 L106 L108 L109 L110 L111 L112 L113 L114 L116 L118 L119 L120 L121 L122 L123 L124 L125 L126 L127 L128 L129 L130 L131 L132 L133 L134 L135 L136 L137 L138 L139 L140 L141 L142 L143 L144 L145 L146 L147 L148 L149 L151 L153 L155 L156 L157 L158 L160 L162 L164 L165 L166 L167 L168 L169 L170 L171 L172 L173 L174 L175 L176 L177 L178 L179 L180 L181 L182 L183 L184 L185 L186 L187 L188 L189 L190 L191 L192 L193 L194 L196 L198 L200 L201 L202 L203 L204 L206 L208 L209 L210 L211 L212 L213 L214 L215 L216 L217 L218 L219 L220 L221 L222 L223 L224 L225 L226 L227 L228 L229 L230 L231 L232 L233 L234 L235 L236 L237 L238 L239 L241 L243 L244 L245 L246 L247 L248 L249 L251 L253 L254 L255 L256 L257 L258 L259 L260 L261 L262 L263 L264 L265 L266 L267 L268 L269 L270 L271 L272 L273 L274 L275 L276 L277 L278 L279 L280 L281 L282 L283 L284 L286 L288 L290 L291 L292 L293 L295 L297 L299 L300 L301 L302 L303 L304 L305 L306 L307 L308 L309 L310 L311 L312 L313 L314 L315 L316 L317 L318 L319 L320 L321 L322 L323 L324 L325 L326 L327 L328 L329 L331 L333 L335 L336 L337 L338 L339 L341 L343 L344 L345 L346 L347 L348 L349 L350 L351 L352 L353 L354 L355 L356 L357 L358 L359 L360 L361 L362 L363 L364 L365 L366 L367 L368 L369 L370 L371 L372 L373 L374 L376 L378 L379 L380 L381 L382 L383 L385 L387 L389 L390 L391 L392 L393 L394 L395 L396 L397 L398 L399 L400 L401 L402 L403 L404 L405 L406 L407 L408 L409 L410 L411 L412 L413 L414 L415 L416 L417 L418 L419 L421 L423 L425 L426 L427 L428 L430 L432 L434 L435 L436 L437 L438 L439 L440 L441 L442 L443 L444 L445 L446 L447 L448 L449 L450 L451 L452 L453 L454 L455 L456 L457 L458 L459 L460 L461 L462 L463 L464 L466 L468 L470 L471 L472 L473 L474 L476 L478 L479 L480 L481 L482 L483 L484 L485 L486 L487 L488 L489 L490 L491 L492 L493 L494 L495 L496 L497 L498 L499 L500 L501 L502 L503 L504 L505 L506 L507 L508 L509 L511 L513 L514 L515 L516 L517 L518 L520 L522 L524 L525 L526 L527 L528 L529 L530 L531 L532 L533 L534 L535 L536 L537 L538 L539 L540 L541 L542 L543 L544 L545 L546 L547 L548 L549 L550 L551 L552 L553 L554 L556 L558 L560 L561 L562 L563 | A0
extrude "Extrusion2" cut sketch "Sketch1" along normal blind 10 contours A0
sketch "Sketch2" plane through (0, 0, 0) normal (0, -1, 0) x (1, 0, 0)
  circle A0 centre (-0.3799, 0.3799) radius 0.057
  circle A1 centre (-0.3799, 0.3799) radius 0.057
  line L0 (-0.0835, 0.3886) -> (-0.0821, 0.3902)
  line L1 (-0.0821, 0.3902) -> (-0.0807, 0.3913)
  line L2 (-0.0807, 0.3913) -> (-0.0794, 0.3923)
  line L3 (-0.0794, 0.3923) -> (-0.078, 0.393)
  line L4 (-0.078, 0.393) -> (-0.0766, 0.3937)
  line L5 (-0.0766, 0.3937) -> (-0.0738, 0.3947)
  line L6 (-0.0738, 0.3947) -> (-0.071, 0.3955)
  line L7 (-0.071, 0.3955) -> (-0.0682, 0.396)
  line L8 (-0.0682, 0.396) -> (-0.0626, 0.3967)
  line L9 (-0.0626, 0.3967) -> (-0.057, 0.3978)
  line L10 (-0.057, 0.3978) -> (-0.0514, 0.3995)
  line L11 (-0.0514, 0.3995) -> (-0.0459, 0.4016)
  line L12 (-0.0459, 0.4016) -> (-0.0404, 0.404)
  line L13 (-0.0404, 0.404) -> (-0.035, 0.4068)
  line L14 (-0.035, 0.4068) -> (-0.0295, 0.4098)
  line L15 (-0.0295, 0.4098) -> (-0.0242, 0.4131)
  line L16 (-0.0242, 0.4131) -> (-0.0188, 0.4167)
  line L17 (-0.0188, 0.4167) -> (-0.0136, 0.4206)
  line L18 (-0.0136, 0.4206) -> (-0.0083, 0.4246)
  line L19 (-0.0083, 0.4246) -> (-0.0032, 0.4289)
  line L20 (-0.0032, 0.4289) -> (-0.0136, 0.4806)
  line L21 (-0.0136, 0.4806) -> (-0.02, 0.4826)
  line L22 (-0.02, 0.4826) -> (-0.0264, 0.4844)
  line L23 (-0.0264, 0.4844) -> (-0.0328, 0.4858)
  line L24 (-0.0328, 0.4858) -> (-0.0391, 0.4871)
  line L25 (-0.0391, 0.4871) -> (-0.0453, 0.488)
  line L26 (-0.0453, 0.488) -> (-0.0515, 0.4888)
  line L27 (-0.0515, 0.4888) -> (-0.0576, 0.4892)
  line L28 (-0.0576, 0.4892) -> (-0.0636, 0.4893)
  line L29 (-0.0636, 0.4893) -> (-0.0695, 0.4891)
  line L30 (-0.0695, 0.4891) -> (-0.0753, 0.4885)
  line L31 (-0.0753, 0.4885) -> (-0.0809, 0.4873)
  line L32 (-0.0809, 0.4873) -> (-0.0863, 0.4858)
  line L33 (-0.0863, 0.4858) -> (-0.0891, 0.4852)
  line L34 (-0.0891, 0.4852) -> (-0.092, 0.4848)
  line L35 (-0.092, 0.4848) -> (-0.095, 0.4847)
  line L36 (-0.095, 0.4847) -> (-0.0965, 0.4848)
  line L37 (-0.0965, 0.4848) -> (-0.0981, 0.4849)
  line L38 (-0.0981, 0.4849) -> (-0.0997, 0.4852)
  line L39 (-0.0997, 0.4852) -> (-0.1014, 0.4858)
  line L40 (-0.1014, 0.4858) -> (-0.1033, 0.4867)
  line L41 (-0.1033, 0.4867) -> (-0.106, 0.4899)
  line L42 (-0.106, 0.4899) -> (-0.1155, 0.5111)
  line L43 (-0.1155, 0.5111) -> (-0.1267, 0.5315)
  line L44 (-0.1267, 0.5315) -> (-0.1275, 0.5356)
  line L45 (-0.1275, 0.5356) -> (-0.1272, 0.5377)
  line L46 (-0.1272, 0.5377) -> (-0.1265, 0.5394)
  line L47 (-0.1265, 0.5394) -> (-0.1258, 0.5409)
  line L48 (-0.1258, 0.5409) -> (-0.125, 0.5422)
  line L49 (-0.125, 0.5422) -> (-0.1241, 0.5435)
  line L50 (-0.1241, 0.5435) -> (-0.1222, 0.5457)
  line L51 (-0.1222, 0.5457) -> (-0.1202, 0.5478)
  line L52 (-0.1202, 0.5478) -> (-0.1181, 0.5497)
  line L53 (-0.1181, 0.5497) -> (-0.1135, 0.5531)
  line L54 (-0.1135, 0.5531) -> (-0.1092, 0.5568)
  line L55 (-0.1092, 0.5568) -> (-0.1052, 0.5611)
  line L56 (-0.1052, 0.5611) -> (-0.1015, 0.5657)
  line L57 (-0.1015, 0.5657) -> (-0.098, 0.5705)
  line L58 (-0.098, 0.5705) -> (-0.0946, 0.5756)
  line L59 (-0.0946, 0.5756) -> (-0.0914, 0.581)
  line L60 (-0.0914, 0.581) -> (-0.0884, 0.5866)
  line L61 (-0.0884, 0.5866) -> (-0.0856, 0.5923)
  line L62 (-0.0856, 0.5923) -> (-0.083, 0.5983)
  line L63 (-0.083, 0.5983) -> (-0.0805, 0.6044)
  line L64 (-0.0805, 0.6044) -> (-0.0782, 0.6107)
  line L65 (-0.0782, 0.6107) -> (-0.1131, 0.6503)
  line L66 (-0.1131, 0.6503) -> (-0.1196, 0.6488)
  line L67 (-0.1196, 0.6488) -> (-0.126, 0.6471)
  line L68 (-0.126, 0.6471) -> (-0.1323, 0.6452)
  line L69 (-0.1323, 0.6452) -> (-0.1383, 0.6431)
  line L70 (-0.1383, 0.6431) -> (-0.1442, 0.6409)
  line L71 (-0.1442, 0.6409) -> (-0.1499, 0.6384)
  line L72 (-0.1499, 0.6384) -> (-0.1554, 0.6357)
  line L73 (-0.1554, 0.6357) -> (-0.1607, 0.6328)
  line L74 (-0.1607, 0.6328) -> (-0.1657, 0.6296)
  line L75 (-0.1657, 0.6296) -> (-0.1704, 0.6262)
  line L76 (-0.1704, 0.6262) -> (-0.1747, 0.6224)
  line L77 (-0.1747, 0.6224) -> (-0.1786, 0.6184)
  line L78 (-0.1786, 0.6184) -> (-0.1807, 0.6165)
  line L79 (-0.1807, 0.6165) -> (-0.183, 0.6147)
  line L80 (-0.183, 0.6147) -> (-0.1855, 0.6131)
  line L81 (-0.1855, 0.6131) -> (-0.1869, 0.6124)
  line L82 (-0.1869, 0.6124) -> (-0.1883, 0.6118)
  line L83 (-0.1883, 0.6118) -> (-0.1899, 0.6112)
  line L84 (-0.1899, 0.6112) -> (-0.1917, 0.6108)
  line L85 (-0.1917, 0.6108) -> (-0.1937, 0.6107)
  line L86 (-0.1937, 0.6107) -> (-0.1978, 0.6121)
  line L87 (-0.1978, 0.6121) -> (-0.2166, 0.6257)
  line L88 (-0.2166, 0.6257) -> (-0.2364, 0.6378)
  line L89 (-0.2364, 0.6378) -> (-0.2392, 0.6409)
  line L90 (-0.2392, 0.6409) -> (-0.2399, 0.6429)
  line L91 (-0.2399, 0.6429) -> (-0.2402, 0.6447)
  line L92 (-0.2402, 0.6447) -> (-0.2403, 0.6463)
  line L93 (-0.2403, 0.6463) -> (-0.2403, 0.6479)
  line L94 (-0.2403, 0.6479) -> (-0.2402, 0.6494)
  line L95 (-0.2402, 0.6494) -> (-0.2397, 0.6524)
  line L96 (-0.2397, 0.6524) -> (-0.2389, 0.6552)
  line L97 (-0.2389, 0.6552) -> (-0.238, 0.6579)
  line L98 (-0.238, 0.6579) -> (-0.2358, 0.6631)
  line L99 (-0.2358, 0.6631) -> (-0.234, 0.6685)
  line L100 (-0.234, 0.6685) -> (-0.2326, 0.6741)
  line L101 (-0.2326, 0.6741) -> (-0.2317, 0.68)
  line L102 (-0.2317, 0.68) -> (-0.2311, 0.6859)
  line L103 (-0.2311, 0.6859) -> (-0.2307, 0.6921)
  line L104 (-0.2307, 0.6921) -> (-0.2306, 0.6983)
  line L105 (-0.2306, 0.6983) -> (-0.2308, 0.7046)
  line L106 (-0.2308, 0.7046) -> (-0.2312, 0.711)
  line L107 (-0.2312, 0.711) -> (-0.2319, 0.7175)
  line L108 (-0.2319, 0.7175) -> (-0.2328, 0.724)
  line L109 (-0.2328, 0.724) -> (-0.234, 0.7306)
  line L110 (-0.234, 0.7306) -> (-0.284, 0.7475)
  line L111 (-0.284, 0.7475) -> (-0.2889, 0.7429)
  line L112 (-0.2889, 0.7429) -> (-0.2936, 0.7382)
  line L113 (-0.2936, 0.7382) -> (-0.2981, 0.7335)
  line L114 (-0.2981, 0.7335) -> (-0.3023, 0.7286)
  line L115 (-0.3023, 0.7286) -> (-0.3063, 0.7237)
  line L116 (-0.3063, 0.7237) -> (-0.31, 0.7187)
  line L117 (-0.31, 0.7187) -> (-0.3134, 0.7137)
  line L118 (-0.3134, 0.7137) -> (-0.3165, 0.7085)
  line L119 (-0.3165, 0.7085) -> (-0.3193, 0.7033)
  line L120 (-0.3193, 0.7033) -> (-0.3216, 0.698)
  line L121 (-0.3216, 0.698) -> (-0.3234, 0.6926)
  line L122 (-0.3234, 0.6926) -> (-0.3248, 0.6871)
  line L123 (-0.3248, 0.6871) -> (-0.3257, 0.6844)
  line L124 (-0.3257, 0.6844) -> (-0.3268, 0.6817)
  line L125 (-0.3268, 0.6817) -> (-0.3282, 0.6791)
  line L126 (-0.3282, 0.6791) -> (-0.329, 0.6778)
  line L127 (-0.329, 0.6778) -> (-0.3299, 0.6765)
  line L128 (-0.3299, 0.6765) -> (-0.331, 0.6752)
  line L129 (-0.331, 0.6752) -> (-0.3323, 0.674)
  line L130 (-0.3323, 0.674) -> (-0.3341, 0.6729)
  line L131 (-0.3341, 0.6729) -> (-0.3382, 0.6721)
  line L132 (-0.3382, 0.6721) -> (-0.3613, 0.6744)
  line L133 (-0.3613, 0.6744) -> (-0.3846, 0.675)
  line L134 (-0.3846, 0.675) -> (-0.3886, 0.6763)
  line L135 (-0.3886, 0.6763) -> (-0.3902, 0.6777)
  line L136 (-0.3902, 0.6777) -> (-0.3913, 0.679)
  line L137 (-0.3913, 0.679) -> (-0.3923, 0.6804)
  line L138 (-0.3923, 0.6804) -> (-0.393, 0.6818)
  line L139 (-0.393, 0.6818) -> (-0.3937, 0.6832)
  line L140 (-0.3937, 0.6832) -> (-0.3947, 0.686)
  line L141 (-0.3947, 0.686) -> (-0.3955, 0.6887)
  line L142 (-0.3955, 0.6887) -> (-0.396, 0.6915)
  line L143 (-0.396, 0.6915) -> (-0.3967, 0.6972)
  line L144 (-0.3967, 0.6972) -> (-0.3978, 0.7028)
  line L145 (-0.3978, 0.7028) -> (-0.3995, 0.7083)
  line L146 (-0.3995, 0.7083) -> (-0.4016, 0.7139)
  line L147 (-0.4016, 0.7139) -> (-0.404, 0.7194)
  line L148 (-0.404, 0.7194) -> (-0.4068, 0.7248)
  line L149 (-0.4068, 0.7248) -> (-0.4098, 0.7302)
  line L150 (-0.4098, 0.7302) -> (-0.4131, 0.7356)
  line L151 (-0.4131, 0.7356) -> (-0.4167, 0.7409)
  line L152 (-0.4167, 0.7409) -> (-0.4205, 0.7462)
  line L153 (-0.4205, 0.7462) -> (-0.4246, 0.7514)
  line L154 (-0.4246, 0.7514) -> (-0.4289, 0.7566)
  line L155 (-0.4289, 0.7566) -> (-0.4806, 0.7462)
  line L156 (-0.4806, 0.7462) -> (-0.4826, 0.7397)
  line L157 (-0.4826, 0.7397) -> (-0.4843, 0.7334)
  line L158 (-0.4843, 0.7334) -> (-0.4858, 0.727)
  line L159 (-0.4858, 0.727) -> (-0.4871, 0.7207)
  line L160 (-0.4871, 0.7207) -> (-0.488, 0.7145)
  line L161 (-0.488, 0.7145) -> (-0.4887, 0.7083)
  line L162 (-0.4887, 0.7083) -> (-0.4892, 0.7022)
  line L163 (-0.4892, 0.7022) -> (-0.4893, 0.6962)
  line L164 (-0.4893, 0.6962) -> (-0.4891, 0.6903)
  line L165 (-0.4891, 0.6903) -> (-0.4885, 0.6845)
  line L166 (-0.4885, 0.6845) -> (-0.4873, 0.6789)
  line L167 (-0.4873, 0.6789) -> (-0.4858, 0.6734)
  line L168 (-0.4858, 0.6734) -> (-0.4852, 0.6706)
  line L169 (-0.4852, 0.6706) -> (-0.4848, 0.6678)
  line L170 (-0.4848, 0.6678) -> (-0.4847, 0.6648)
  line L171 (-0.4847, 0.6648) -> (-0.4848, 0.6633)
  line L172 (-0.4848, 0.6633) -> (-0.4849, 0.6617)
  line L173 (-0.4849, 0.6617) -> (-0.4852, 0.6601)
  line L174 (-0.4852, 0.6601) -> (-0.4858, 0.6584)
  line L175 (-0.4858, 0.6584) -> (-0.4867, 0.6565)
  line L176 (-0.4867, 0.6565) -> (-0.4899, 0.6537)
  line L177 (-0.4899, 0.6537) -> (-0.5111, 0.6442)
  line L178 (-0.5111, 0.6442) -> (-0.5315, 0.6331)
  line L179 (-0.5315, 0.6331) -> (-0.5356, 0.6322)
  line L180 (-0.5356, 0.6322) -> (-0.5377, 0.6326)
  line L181 (-0.5377, 0.6326) -> (-0.5394, 0.6332)
  line L182 (-0.5394, 0.6332) -> (-0.5409, 0.634)
  line L183 (-0.5409, 0.634) -> (-0.5422, 0.6348)
  line L184 (-0.5422, 0.6348) -> (-0.5435, 0.6356)
  line L185 (-0.5435, 0.6356) -> (-0.5457, 0.6375)
  line L186 (-0.5457, 0.6375) -> (-0.5478, 0.6396)
  line L187 (-0.5478, 0.6396) -> (-0.5497, 0.6417)
  line L188 (-0.5497, 0.6417) -> (-0.5531, 0.6463)
  line L189 (-0.5531, 0.6463) -> (-0.5568, 0.6505)
  line L190 (-0.5568, 0.6505) -> (-0.5611, 0.6545)
  line L191 (-0.5611, 0.6545) -> (-0.5657, 0.6583)
  line L192 (-0.5657, 0.6583) -> (-0.5705, 0.6618)
  line L193 (-0.5705, 0.6618) -> (-0.5756, 0.6652)
  line L194 (-0.5756, 0.6652) -> (-0.581, 0.6683)
  line L195 (-0.581, 0.6683) -> (-0.5865, 0.6713)
  line L196 (-0.5865, 0.6713) -> (-0.5923, 0.6742)
  line L197 (-0.5923, 0.6742) -> (-0.5983, 0.6768)
  line L198 (-0.5983, 0.6768) -> (-0.6044, 0.6793)
  line L199 (-0.6044, 0.6793) -> (-0.6107, 0.6816)
  line L200 (-0.6107, 0.6816) -> (-0.6503, 0.6467)
  line L201 (-0.6503, 0.6467) -> (-0.6488, 0.6402)
  line L202 (-0.6488, 0.6402) -> (-0.6471, 0.6338)
  line L203 (-0.6471, 0.6338) -> (-0.6452, 0.6275)
  line L204 (-0.6452, 0.6275) -> (-0.6431, 0.6214)
  line L205 (-0.6431, 0.6214) -> (-0.6408, 0.6156)
  line L206 (-0.6408, 0.6156) -> (-0.6384, 0.6099)
  line L207 (-0.6384, 0.6099) -> (-0.6357, 0.6044)
  line L208 (-0.6357, 0.6044) -> (-0.6328, 0.5991)
  line L209 (-0.6328, 0.5991) -> (-0.6296, 0.5941)
  line L210 (-0.6296, 0.5941) -> (-0.6262, 0.5894)
  line L211 (-0.6262, 0.5894) -> (-0.6224, 0.5851)
  line L212 (-0.6224, 0.5851) -> (-0.6184, 0.5812)
  line L213 (-0.6184, 0.5812) -> (-0.6165, 0.579)
  line L214 (-0.6165, 0.579) -> (-0.6147, 0.5767)
  line L215 (-0.6147, 0.5767) -> (-0.6131, 0.5742)
  line L216 (-0.6131, 0.5742) -> (-0.6124, 0.5729)
  line L217 (-0.6124, 0.5729) -> (-0.6118, 0.5714)
  line L218 (-0.6118, 0.5714) -> (-0.6112, 0.5699)
  line L219 (-0.6112, 0.5699) -> (-0.6108, 0.5681)
  line L220 (-0.6108, 0.5681) -> (-0.6107, 0.566)
  line L221 (-0.6107, 0.566) -> (-0.6121, 0.562)
  line L222 (-0.6121, 0.562) -> (-0.6257, 0.5432)
  line L223 (-0.6257, 0.5432) -> (-0.6378, 0.5234)
  line L224 (-0.6378, 0.5234) -> (-0.6409, 0.5205)
  line L225 (-0.6409, 0.5205) -> (-0.6429, 0.5198)
  line L226 (-0.6429, 0.5198) -> (-0.6447, 0.5195)
  line L227 (-0.6447, 0.5195) -> (-0.6463, 0.5194)
  line L228 (-0.6463, 0.5194) -> (-0.6479, 0.5195)
  line L229 (-0.6479, 0.5195) -> (-0.6494, 0.5196)
  line L230 (-0.6494, 0.5196) -> (-0.6523, 0.5201)
  line L231 (-0.6523, 0.5201) -> (-0.6551, 0.5208)
  line L232 (-0.6551, 0.5208) -> (-0.6578, 0.5217)
  line L233 (-0.6578, 0.5217) -> (-0.6631, 0.524)
  line L234 (-0.6631, 0.524) -> (-0.6685, 0.5258)
  line L235 (-0.6685, 0.5258) -> (-0.6741, 0.5271)
  line L236 (-0.6741, 0.5271) -> (-0.68, 0.5281)
  line L237 (-0.68, 0.5281) -> (-0.6859, 0.5287)
  line L238 (-0.6859, 0.5287) -> (-0.692, 0.5291)
  line L239 (-0.692, 0.5291) -> (-0.6983, 0.5291)
  line L240 (-0.6983, 0.5291) -> (-0.7046, 0.529)
  line L241 (-0.7046, 0.529) -> (-0.711, 0.5285)
  line L242 (-0.711, 0.5285) -> (-0.7175, 0.5278)
  line L243 (-0.7175, 0.5278) -> (-0.724, 0.5269)
  line L244 (-0.724, 0.5269) -> (-0.7306, 0.5258)
  line L245 (-0.7306, 0.5258) -> (-0.7475, 0.4758)
  line L246 (-0.7475, 0.4758) -> (-0.7429, 0.4708)
  line L247 (-0.7429, 0.4708) -> (-0.7382, 0.4661)
  line L248 (-0.7382, 0.4661) -> (-0.7335, 0.4617)
  line L249 (-0.7335, 0.4617) -> (-0.7286, 0.4575)
  line L250 (-0.7286, 0.4575) -> (-0.7237, 0.4535)
  line L251 (-0.7237, 0.4535) -> (-0.7187, 0.4498)
  line L252 (-0.7187, 0.4498) -> (-0.7137, 0.4464)
  line L253 (-0.7137, 0.4464) -> (-0.7085, 0.4433)
  line L254 (-0.7085, 0.4433) -> (-0.7033, 0.4405)
  line L255 (-0.7033, 0.4405) -> (-0.698, 0.4381)
  line L256 (-0.698, 0.4381) -> (-0.6926, 0.4363)
  line L257 (-0.6926, 0.4363) -> (-0.6871, 0.4349)
  line L258 (-0.6871, 0.4349) -> (-0.6844, 0.434)
  line L259 (-0.6844, 0.434) -> (-0.6817, 0.4329)
  line L260 (-0.6817, 0.4329) -> (-0.6791, 0.4316)
  line L261 (-0.6791, 0.4316) -> (-0.6778, 0.4308)
  line L262 (-0.6778, 0.4308) -> (-0.6765, 0.4298)
  line L263 (-0.6765, 0.4298) -> (-0.6752, 0.4287)
  line L264 (-0.6752, 0.4287) -> (-0.674, 0.4274)
  line L265 (-0.674, 0.4274) -> (-0.6729, 0.4257)
  line L266 (-0.6729, 0.4257) -> (-0.6721, 0.4215)
  line L267 (-0.6721, 0.4215) -> (-0.6744, 0.3984)
  line L268 (-0.6744, 0.3984) -> (-0.675, 0.3752)
  line L269 (-0.675, 0.3752) -> (-0.6763, 0.3712)
  line L270 (-0.6763, 0.3712) -> (-0.6777, 0.3696)
  line L271 (-0.6777, 0.3696) -> (-0.679, 0.3684)
  line L272 (-0.679, 0.3684) -> (-0.6804, 0.3675)
  line L273 (-0.6804, 0.3675) -> (-0.6818, 0.3667)
  line L274 (-0.6818, 0.3667) -> (-0.6832, 0.3661)
  line L275 (-0.6832, 0.3661) -> (-0.686, 0.3651)
  line L276 (-0.686, 0.3651) -> (-0.6887, 0.3643)
  line L277 (-0.6887, 0.3643) -> (-0.6915, 0.3637)
  line L278 (-0.6915, 0.3637) -> (-0.6972, 0.3631)
  line L279 (-0.6972, 0.3631) -> (-0.7028, 0.3619)
  line L280 (-0.7028, 0.3619) -> (-0.7083, 0.3603)
  line L281 (-0.7083, 0.3603) -> (-0.7139, 0.3582)
  line L282 (-0.7139, 0.3582) -> (-0.7194, 0.3557)
  line L283 (-0.7194, 0.3557) -> (-0.7248, 0.353)
  line L284 (-0.7248, 0.353) -> (-0.7302, 0.3499)
  line L285 (-0.7302, 0.3499) -> (-0.7356, 0.3466)
  line L286 (-0.7356, 0.3466) -> (-0.7409, 0.343)
  line L287 (-0.7409, 0.343) -> (-0.7462, 0.3392)
  line L288 (-0.7462, 0.3392) -> (-0.7514, 0.3351)
  line L289 (-0.7514, 0.3351) -> (-0.7566, 0.3308)
  line L290 (-0.7566, 0.3308) -> (-0.7462, 0.2791)
  line L291 (-0.7462, 0.2791) -> (-0.7397, 0.2771)
  line L292 (-0.7397, 0.2771) -> (-0.7334, 0.2754)
  line L293 (-0.7334, 0.2754) -> (-0.727, 0.2739)
  line L294 (-0.727, 0.2739) -> (-0.7207, 0.2727)
  line L295 (-0.7207, 0.2727) -> (-0.7145, 0.2717)
  line L296 (-0.7145, 0.2717) -> (-0.7083, 0.271)
  line L297 (-0.7083, 0.271) -> (-0.7022, 0.2706)
  line L298 (-0.7022, 0.2706) -> (-0.6962, 0.2705)
  line L299 (-0.6962, 0.2705) -> (-0.6903, 0.2707)
  line L300 (-0.6903, 0.2707) -> (-0.6845, 0.2713)
  line L301 (-0.6845, 0.2713) -> (-0.6789, 0.2724)
  line L302 (-0.6789, 0.2724) -> (-0.6734, 0.274)
  line L303 (-0.6734, 0.274) -> (-0.6706, 0.2746)
  line L304 (-0.6706, 0.2746) -> (-0.6678, 0.2749)
  line L305 (-0.6678, 0.2749) -> (-0.6648, 0.2751)
  line L306 (-0.6648, 0.2751) -> (-0.6633, 0.275)
  line L307 (-0.6633, 0.275) -> (-0.6617, 0.2748)
  line L308 (-0.6617, 0.2748) -> (-0.6601, 0.2745)
  line L309 (-0.6601, 0.2745) -> (-0.6584, 0.274)
  line L310 (-0.6584, 0.274) -> (-0.6565, 0.2731)
  line L311 (-0.6565, 0.2731) -> (-0.6537, 0.2699)
  line L312 (-0.6537, 0.2699) -> (-0.6442, 0.2487)
  line L313 (-0.6442, 0.2487) -> (-0.6331, 0.2283)
  line L314 (-0.6331, 0.2283) -> (-0.6322, 0.2241)
  line L315 (-0.6322, 0.2241) -> (-0.6326, 0.2221)
  line L316 (-0.6326, 0.2221) -> (-0.6332, 0.2204)
  line L317 (-0.6332, 0.2204) -> (-0.634, 0.2189)
  line L318 (-0.634, 0.2189) -> (-0.6348, 0.2176)
  line L319 (-0.6348, 0.2176) -> (-0.6356, 0.2163)
  line L320 (-0.6356, 0.2163) -> (-0.6375, 0.214)
  line L321 (-0.6375, 0.214) -> (-0.6396, 0.212)
  line L322 (-0.6396, 0.212) -> (-0.6417, 0.2101)
  line L323 (-0.6417, 0.2101) -> (-0.6463, 0.2067)
  line L324 (-0.6463, 0.2067) -> (-0.6505, 0.2029)
  line L325 (-0.6505, 0.2029) -> (-0.6545, 0.1987)
  line L326 (-0.6545, 0.1987) -> (-0.6583, 0.1941)
  line L327 (-0.6583, 0.1941) -> (-0.6618, 0.1892)
  line L328 (-0.6618, 0.1892) -> (-0.6652, 0.1841)
  line L329 (-0.6652, 0.1841) -> (-0.6683, 0.1788)
  line L330 (-0.6683, 0.1788) -> (-0.6713, 0.1732)
  line L331 (-0.6713, 0.1732) -> (-0.6742, 0.1675)
  line L332 (-0.6742, 0.1675) -> (-0.6768, 0.1615)
  line L333 (-0.6768, 0.1615) -> (-0.6793, 0.1554)
  line L334 (-0.6793, 0.1554) -> (-0.6816, 0.1491)
  line L335 (-0.6816, 0.1491) -> (-0.6467, 0.1095)
  line L336 (-0.6467, 0.1095) -> (-0.6402, 0.111)
  line L337 (-0.6402, 0.111) -> (-0.6338, 0.1127)
  line L338 (-0.6338, 0.1127) -> (-0.6275, 0.1146)
  line L339 (-0.6275, 0.1146) -> (-0.6214, 0.1166)
  line L340 (-0.6214, 0.1166) -> (-0.6156, 0.1189)
  line L341 (-0.6156, 0.1189) -> (-0.6099, 0.1214)
  line L342 (-0.6099, 0.1214) -> (-0.6044, 0.1241)
  line L343 (-0.6044, 0.1241) -> (-0.5991, 0.127)
  line L344 (-0.5991, 0.127) -> (-0.5941, 0.1301)
  line L345 (-0.5941, 0.1301) -> (-0.5894, 0.1335)
  line L346 (-0.5894, 0.1335) -> (-0.5851, 0.1373)
  line L347 (-0.5851, 0.1373) -> (-0.5812, 0.1414)
  line L348 (-0.5812, 0.1414) -> (-0.579, 0.1433)
  line L349 (-0.579, 0.1433) -> (-0.5767, 0.145)
  line L350 (-0.5767, 0.145) -> (-0.5742, 0.1466)
  line L351 (-0.5742, 0.1466) -> (-0.5729, 0.1474)
  line L352 (-0.5729, 0.1474) -> (-0.5714, 0.148)
  line L353 (-0.5714, 0.148) -> (-0.5699, 0.1485)
  line L354 (-0.5699, 0.1485) -> (-0.5681, 0.1489)
  line L355 (-0.5681, 0.1489) -> (-0.566, 0.1491)
  line L356 (-0.566, 0.1491) -> (-0.562, 0.1477)
  line L357 (-0.562, 0.1477) -> (-0.5432, 0.1341)
  line L358 (-0.5432, 0.1341) -> (-0.5234, 0.122)
  line L359 (-0.5234, 0.122) -> (-0.5205, 0.1188)
  line L360 (-0.5205, 0.1188) -> (-0.5198, 0.1169)
  line L361 (-0.5198, 0.1169) -> (-0.5195, 0.1151)
  line L362 (-0.5195, 0.1151) -> (-0.5194, 0.1134)
  line L363 (-0.5194, 0.1134) -> (-0.5194, 0.1119)
  line L364 (-0.5194, 0.1119) -> (-0.5196, 0.1103)
  line L365 (-0.5196, 0.1103) -> (-0.5201, 0.1074)
  line L366 (-0.5201, 0.1074) -> (-0.5208, 0.1046)
  line L367 (-0.5208, 0.1046) -> (-0.5217, 0.1019)
  line L368 (-0.5217, 0.1019) -> (-0.524, 0.0967)
  line L369 (-0.524, 0.0967) -> (-0.5258, 0.0913)
  line L370 (-0.5258, 0.0913) -> (-0.5271, 0.0856)
  line L371 (-0.5271, 0.0856) -> (-0.5281, 0.0798)
  line L372 (-0.5281, 0.0798) -> (-0.5287, 0.0738)
  line L373 (-0.5287, 0.0738) -> (-0.5291, 0.0677)
  line L374 (-0.5291, 0.0677) -> (-0.5291, 0.0615)
  line L375 (-0.5291, 0.0615) -> (-0.529, 0.0552)
  line L376 (-0.529, 0.0552) -> (-0.5285, 0.0488)
  line L377 (-0.5285, 0.0488) -> (-0.5278, 0.0423)
  line L378 (-0.5278, 0.0423) -> (-0.5269, 0.0357)
  line L379 (-0.5269, 0.0357) -> (-0.5258, 0.0291)